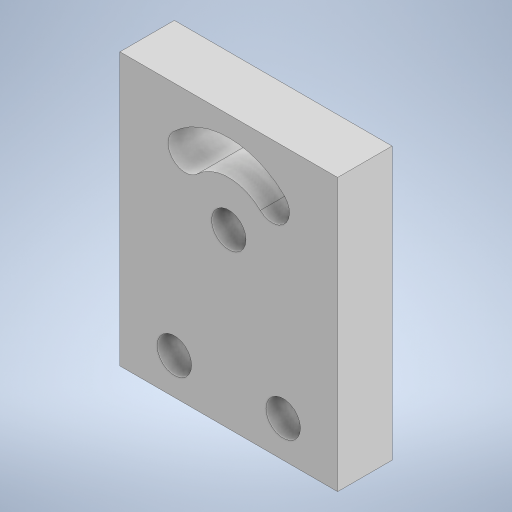
# Autodesk Inventor part: arm_camera_adapter
Saved by Autodesk Inventor 2024 (Build 280153000, 153)
## iProperties
Created: 2023-10-26
Part Number: arm_camera_adapter
Material: Generic
Document SubType Name: Modeling
Designer: dimademler
Density: 1 g/cm^3
Appearance: Default
Author: dimademler
Autodesk Inventor part; units mm, degrees
ref_plane "YZ Plane" through (0, 0, 0) normal (1, 0, 0) x (0, 1, 0)
ref_plane "XZ Plane" through (0, 0, 0) normal (0, 1, 0) x (-1, 0, 0)
ref_plane "XY Plane" through (0, 0, 0) normal (0, 0, 1) x (1, 0, 0)
sketch "Sketch1" plane through (0, 0, 0) normal (0, 0, 1) x (1, 0, 0)
  line L0 (0, 0) -> (30.48, 0)
  line L1 (30.48, 0) -> (30.48, 38.1)
  line L2 (30.48, 38.1) -> (0, 38.1)
  line L3 (0, 38.1) -> (0, 0)
  dimension "d0" = 30.48
  dimension "d1" = 38.1
  constraints: 8 end point, 2 parallel, 1 horizontal, 1 perpendicular
  measures "d0" distance of L0.start L0.end
  measures "d1" distance of L1.end L0.end
extrude "Extrusion1" add sketch "Sketch1" along normal blind 7.62
sketch "Sketch2" plane through (0, 0, 7.62) normal (0, 0, 1) x (1, 0, 0)
  line L0 (0, 0) -> (30.48, 0) projected
  line L1 (0, 38.1) -> (0, 0) projected
  line L2 (30.48, 0) -> (30.48, 38.1) projected
  line L3 (15.24, 0) -> (15.24, 5.08) construction
  line L4 (15.24, 5.08) -> (7.62, 5.08) construction
  circle A0 centre (7.62, 5.08) radius 2.413
  line L5 (15.24, 5.08) -> (22.86, 5.08) construction
  circle A1 centre (22.86, 5.08) radius 2.413
  dimension "d4" = 5.08
  dimension "d5" = 7.62
  dimension "d6" = 4.826
  constraints: 6 end point, 2 centre point, 2 coincident, 2 symmetric about line, 1 horizontal, 1 midpoint, 1 vertical, 1 other
  measures "d4" distance of L3.start L3.end
  measures "d5" distance of L3.end L4.end
  measures "d6" diameter of A0
extrude "Extrusion2" cut sketch "Sketch2" against normal blind 7.62
sketch "Sketch3" plane through (0, 0, 7.62) normal (0, 0, 1) x (1, 0, 0)
  line L0 (0, 38.1) -> (0, 0) projected
  line L1 (30.48, 38.1) -> (0, 38.1) projected
  line L2 (30.48, 0) -> (30.48, 38.1) projected
  line L3 (15.24, 38.1) -> (15.24, 24.13) construction
  circle A0 centre (15.24, 24.13) radius 2.413
  dimension "d9" = 13.97
  dimension "d10" = 4.826
  constraints: 2 end point, 1 centre point, 1 coincident, 1 midpoint, 1 vertical
  measures "d9" distance of L3.start L3.end
  measures "d10" diameter of A0
extrude "Extrusion3" cut sketch "Sketch3" against normal blind 7.62
sketch "Sketch4" plane through (0, 0, 7.62) normal (0, 0, 1) x (1, 0, 0)
  line L0 (0, 38.1) -> (0, 0) projected
  line L1 (30.48, 38.1) -> (0, 38.1) projected
  line L2 (30.48, 0) -> (30.48, 38.1) projected
  circle A0 centre (15.24, 24.13) radius 2.413 projected
  line L3 (15.24, 24.13) -> (15.24, 38.1) construction
  arc A1 (9.7407, 27.305) -> (19.6524, 28.6965) centre (15.24, 24.13) ccw construction
  arc A2 (5.5613, 29.718) -> (23.0058, 32.1671) centre (15.24, 24.13) ccw construction
  line L4 (15.24, 24.13) -> (9.7407, 27.305) construction
  line L5 (15.24, 24.13) -> (25.654, 24.13) construction
  line L6 (15.24, 24.13) -> (20.7393, 27.305) construction
  line L7 (15.24, 24.13) -> (25.654, 24.13) construction
  line L8 (9.7407, 27.305) -> (5.5613, 29.718) construction
  line L9 (20.7393, 27.305) -> (24.9187, 29.718) construction
  arc A3 (7.4742, 32.1671) -> (10.8276, 28.6965) centre (9.1509, 30.4318) ccw
  arc A4 (19.6524, 28.6965) -> (23.0058, 32.1671) centre (21.3291, 30.4318) ccw
  arc A5 (7.4742, 32.1671) -> (5.5613, 29.718) centre (15.24, 24.13) ccw construction
  arc A6 (10.8276, 28.6965) -> (9.7407, 27.305) centre (15.24, 24.13) ccw construction
  arc A7 (19.6524, 28.6965) -> (10.8276, 28.6965) centre (15.24, 24.13) ccw
  arc A8 (23.0058, 32.1671) -> (7.4742, 32.1671) centre (15.24, 24.13) ccw
  arc A9 (23.0058, 32.1671) -> (19.6524, 28.6965) centre (21.3291, 30.4318) ccw construction
  arc A10 (10.8276, 28.6965) -> (7.4742, 32.1671) centre (9.1509, 30.4318) ccw construction
  dimension "d13" = 12.7
  dimension "d14" = 22.352
  dimension "d15" = 150
  dimension "d16" = 30
  dimension "d17" = 4.826
  dimension "d18" = 4.826
  constraints: 24 point on circle, 14 end point, 10 centre point, 4 tangent, 2 coincident, 2 collinear, 2 horizontal, 1 midpoint
  measures "d13" diameter of A1
  measures "d14" diameter of A2
  measures "d15" angle of L5 L4
  measures "d16" angle of L7 L6
  measures "d17" diameter of A3
  measures "d18" diameter of A4
extrude "Extrusion4" cut sketch "Sketch4" against normal through all contours A8 A4 A7 A3
body "Solid1"
